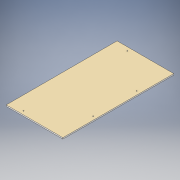
# Autodesk Inventor part: Ceiling 2 Holeless half
Saved by Autodesk Inventor 2017 (Build 210142000, 142)
## iProperties
Created: 2017-07-05
Part Number: Ceiling 2 Holeless half
Material: Generic
Document SubType Name: Modeling
Designer: cas7
Density: 1 g/cm^3
Appearance: Default
Author: cas7
Autodesk Inventor part; units mm, degrees
ref_plane "YZ Plane" through (0, 0, 0) normal (1, 0, 0) x (0, 1, 0)
ref_plane "XZ Plane" through (0, 0, 0) normal (0, 1, 0) x (-1, 0, 0)
ref_plane "XY Plane" through (0, 0, 0) normal (0, 0, 1) x (1, 0, 0)
sketch "Sketch1" plane through (0, 0, 0) normal (0, 1, 0) x (-1, 0, 0)
  line L0 (0, 0) -> (714.375, 0)
  line L1 (714.375, 0) -> (714.375, -1397)
  line L2 (714.375, -1397) -> (0, -1397)
  line L3 (0, -1397) -> (0, 0)
  dimension "d0" = 714.375
  dimension "d1" = 1397
  constraints: 8 end point, 2 parallel, 1 horizontal, 1 perpendicular
  measures "d0" distance of L1.end L2.end
  measures "d1" distance of L0.end L1.end
extrude "Extrusion1" add sketch "Sketch1" along normal blind 15.875
sketch "Sketch2" plane through (0, 15.875, 0) normal (0, 1, 0) x (1, 0, 0)
  line L0 (0, 1397) -> (-714.375, 1397) projected
  line L1 (-714.375, 1397) -> (-714.375, 0) projected
  line L2 (0, 0) -> (-44.45, 0)
  line L3 (0, 0) -> (-714.375, 0) projected
  line L4 (-44.45, 0) -> (-44.45, 425.45)
  line L5 (-44.45, 1397) -> (-44.45, 974.09)
  line L6 (0, 0) -> (-540.5628, 0)
  line L7 (-540.5628, 0) -> (-540.5628, 44.45)
  point P0 (-540.5628, 1352.55)
  dimension "d8" = 44.45
  dimension "d9" = 425.45
  dimension "d10" = 422.91
  dimension "d11" = 540.5628
  constraints: 10 end point, 3 coincident, 3 point on line, 1 parallel, 1 vertical
  measures "d8" distance of L2.start L2.end
  measures "d9" distance of L2.end L4.end
  measures "d10" distance of L5.start L5.end
  measures "d11" distance of L2.start L6.end
hole "Hole1" at (-540.5628, 15.875, -44.45) at (-540.5628, 15.875, -1352.55) at (-44.45, 15.875, -974.09) at (-44.45, 15.875, -425.45) direction (0, -1, 0) diameter 10.5918 depth 35.179 tip angle 118 thread size "1/2-13 UNC" class "2B" standard "ANSI Unified Screw Threads"
body "Solid1"
